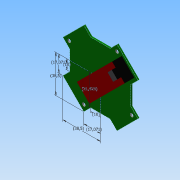
# Autodesk Inventor part: x_board
Saved by Autodesk Inventor 2015 (Build 190159000, 159)
## iProperties
Created: 2015-08-03
Part Number: x_board
Material: Générique
Document SubType Name: Modeling
Designer: Gregwar
Density: 1 g/cm^3
Appearance: Par défaut
Author: Gregwar
Autodesk Inventor part; units mm, degrees
ref_plane "YZ Plane" through (0, 0, 0) normal (1, 0, 0) x (0, 1, 0)
ref_plane "XZ Plane" through (0, 0, 0) normal (0, 1, 0) x (-1, 0, 0)
ref_plane "XY Plane" through (0, 0, 0) normal (0, 0, 1) x (1, 0, 0)
sketch "Esquisse1" plane through (0, 0, 0) normal (0, 1, 0) x (-1, 0, 0)
  line L0 (0, 0) -> (40.8419, 40.8419) construction
  line L1 (0, 0) -> (43.2459, 0) construction
  line L2 (0, 0) -> (0, 37.214) construction
  line L3 (31.4289, 0) -> (31.4289, 10)
  line L4 (31.4289, 10) -> (38.5, 17.0711)
  line L5 (38.5, 17.0711) -> (27.7855, 27.7855)
  line L6 (0, 31.4289) -> (10, 31.4289)
  line L7 (10, 31.4289) -> (17.0711, 38.5)
  line L8 (17.0711, 38.5) -> (27.7855, 27.7855)
  line L9 (31.4289, 0) -> (31.4289, -10)
  line L10 (31.4289, -10) -> (38.5, -17.0711)
  line L11 (38.5, -17.0711) -> (27.7855, -27.7855)
  line L12 (0, -31.4289) -> (10, -31.4289)
  line L13 (10, -31.4289) -> (17.0711, -38.5)
  line L14 (17.0711, -38.5) -> (27.7855, -27.7855)
  line L15 (0, 0) -> (-40.8419, 40.8419) construction
  line L16 (0, 0) -> (-43.2459, 0) construction
  line L17 (-31.4289, 0) -> (-31.4289, 10)
  line L18 (-31.4289, 10) -> (-38.5, 17.0711)
  line L19 (-38.5, 17.0711) -> (-27.7855, 27.7855)
  line L20 (0, 31.4289) -> (-10, 31.4289)
  line L21 (-10, 31.4289) -> (-17.0711, 38.5)
  line L22 (-17.0711, 38.5) -> (-27.7855, 27.7855)
  line L23 (-38.5, -17.0711) -> (-27.7855, -27.7855)
  line L24 (-31.4289, -10) -> (-38.5, -17.0711)
  line L25 (-31.4289, 0) -> (-31.4289, -10)
  line L26 (-17.0711, -38.5) -> (-27.7855, -27.7855)
  line L27 (-10, -31.4289) -> (-17.0711, -38.5)
  line L28 (0, -31.4289) -> (-10, -31.4289)
  dimension "d4" = 45
  dimension "d5" = 10
  dimension "d6" = 10
  dimension "d7" = 38.5
  dimension "d10" = 77
  constraints: 58 end point, 22 symmetric about line, 4 point on line, 2 vertical, 1 collinear, 1 horizontal, 1 parallel
  measures "d4" angle of L0 L1
  measures "d5" distance of L3.start L3.end
  measures "d6" distance of L3.end L4.end
  measures "d7" distance from line of L1 L7.end
  measures "d10" distance of L14.start L7.end
extrude "Extrusion1" add sketch "Esquisse1" along normal blind 1.6
sketch "Esquisse3" plane through (0, 0, 0) normal (0, -1, 0) x (1, 0, 0)
  line L0 (-31.4289, -10) -> (-31.4289, 10) construction
  line L1 (-38.5, -17.0711) -> (-31.4289, -10) construction
  line L2 (-17.0711, -38.5) -> (-38.5, -17.0711) construction
  line L3 (-10, -31.4289) -> (-17.0711, -38.5) construction
  line L4 (10, -31.4289) -> (-10, -31.4289) construction
  line L5 (17.0711, -38.5) -> (10, -31.4289) construction
  line L6 (38.5, -17.0711) -> (17.0711, -38.5) construction
  line L7 (31.4289, -10) -> (38.5, -17.0711) construction
  line L8 (31.4289, 10) -> (31.4289, -10) construction
  line L9 (38.5, 17.0711) -> (31.4289, 10) construction
  line L10 (17.0711, 38.5) -> (38.5, 17.0711) construction
  line L11 (10, 31.4289) -> (17.0711, 38.5) construction
  line L12 (-10, 31.4289) -> (10, 31.4289) construction
  line L13 (-17.0711, 38.5) -> (-10, 31.4289) construction
  line L14 (-38.5, 17.0711) -> (-17.0711, 38.5) construction
  line L15 (-31.4289, 10) -> (-38.5, 17.0711) construction
  circle A0 centre (-32.136, 17.0711) radius 1.75
  circle A1 centre (-17.0711, -32.136) radius 1.75
  circle A2 centre (32.136, -17.0711) radius 1.75
  circle A3 centre (17.0711, 32.136) radius 1.75
  point P0 (0, 0)
  point P1 (16, 32)
  point P2 (0, 0)
  point P3 (0, 0)
  point P4 (0, 0)
  dimension "d36" = 4.5
  dimension "d37" = 4.5
  dimension "d38" = 3.5
  dimension "d41" = 360
  constraints: 4 centre point, 2 coincident, 11 other
  measures "d36" distance from line of L15 A0.centre
  measures "d37" distance from line of L14 A0.centre
  measures "d38" diameter of A0
extrude "Extrusion2" cut sketch "Esquisse3" against normal through all
sketch "Esquisse4" plane through (0, 0, 0) normal (0, -1, 0) x (1, 0, 0)
  point P0 (0, 0)
sketch "Esquisse5" plane through (0, 0, 0) normal (0, -1, 0) x (1, 0, 0)
  line L0 (-31.4289, -10) -> (-31.4289, 10) construction
  line L1 (-38.5, -17.0711) -> (-31.4289, -10) construction
  line L2 (-17.0711, -38.5) -> (-38.5, -17.0711) construction
  line L3 (-10, -31.4289) -> (-17.0711, -38.5) construction
  line L4 (10, -31.4289) -> (-10, -31.4289) construction
  line L5 (17.0711, -38.5) -> (10, -31.4289) construction
  line L6 (38.5, -17.0711) -> (17.0711, -38.5) construction
  line L7 (31.4289, -10) -> (38.5, -17.0711) construction
  line L8 (31.4289, 10) -> (31.4289, -10) construction
  line L9 (38.5, 17.0711) -> (31.4289, 10) construction
  line L10 (17.0711, 38.5) -> (38.5, 17.0711) construction
  line L11 (10, 31.4289) -> (17.0711, 38.5) construction
  line L12 (-10, 31.4289) -> (10, 31.4289) construction
  line L13 (-17.0711, 38.5) -> (-10, 31.4289) construction
  line L14 (-38.5, 17.0711) -> (-17.0711, 38.5) construction
  line L15 (-31.4289, 10) -> (-38.5, 17.0711) construction
  line L16 (0, 0) -> (-31.4289, 0) construction
  line L17 (0, 0) -> (0, -31.4289) construction
  dimension "d29" = 38.5
  dimension "d30" = 17.0711
  dimension "d31" = 31.4289
  dimension "d32" = 10
  dimension "d33" = 17.0711
  dimension "d34" = 38.5
  dimension "d35" = 10
  constraints: 4 end point, 2 midpoint
  measures "d29" distance from line of L2.start L16
  measures "d30" distance from line of L2.start L17
  measures "d31" distance from line of L3.start L16
  measures "d32" distance from line of L17 L3.start
  measures "d33" distance from line of L16 L1.start
  measures "d34" distance from line of L17 L1.start
  measures "d35" distance from line of L0.start L16
sketch "Esquisse6" plane through (0, 0, 0) normal (0, -1, 0) x (1, 0, 0)
  line L0 (22.0329, 30.7097) -> (-14.2473, -5.5705)
  line L1 (-14.2473, -5.5705) -> (-1.3158, -18.5021)
  line L2 (-1.3158, -18.5021) -> (34.9645, 17.7782)
  line L3 (34.9645, 17.7782) -> (22.0329, 30.7097)
  line L4 (17.0711, 38.5) -> (38.5, 17.0711) projected
  line L5 (38.5, 17.0711) -> (31.4289, 10) projected
  point P0 (0, 0)
  dimension "d43" = 2
  dimension "d44" = 51.308
  dimension "d45" = 18.288
  dimension "d46" = 3
  constraints: 8 end point, 2 parallel, 2 perpendicular
  measures "d43" distance between parallel lines of L4 L3
  measures "d44" distance of L1.end L2.end
  measures "d45" distance between parallel lines of L0 L2
  measures "d46" distance between parallel lines of L5 L2
extrude "Extrusion3" add sketch "Esquisse6" along normal blind 10
sketch "Esquisse7" plane through (0, -10, 0) normal (0, -1, 0) x (1, 0, 0)
  line L0 (21.4276, 22.8297) -> (27.0845, 17.1729)
  line L1 (27.0845, 17.1729) -> (31.3271, 21.4155)
  line L2 (31.3271, 21.4155) -> (25.6703, 27.0724)
  line L3 (25.6703, 27.0724) -> (21.4276, 22.8297)
  line L4 (34.9645, 17.7782) -> (22.0329, 30.7097) projected
  point P0 (0, 0)
  point P1 (28.4987, 24.244)
  dimension "d49" = 8
  dimension "d50" = 6
  constraints: 8 end point, 2 midpoint, 2 perpendicular, 1 collinear, 1 parallel
  measures "d49" distance of L0.start L0.end
  measures "d50" distance of L2.end L0.start
extrude "Extrusion4" add sketch "Esquisse7" along normal blind 4
